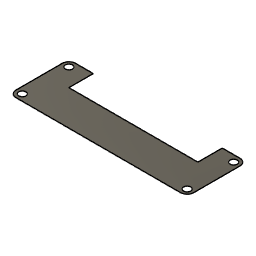
AppleFootToMultiPurposeHolder v1 (Autodesk Fusion 360 design; units mm, degrees)
Autodesk Fusion 360 part; units mm, degrees
sketch "Sketch1" plane through (0, 0, 0) normal (0, 0, 1) x (1, 0, 0)
  line L0 (0, 0) -> (55, 0) construction
  line L1 (0, 0) -> (-55, 0) construction
  circle A0 centre (-57.5, 0) radius 2.5
  circle A1 centre (57.5, 0) radius 2.5
  line L2 (-57.5, -2.5) -> (-57.5, -30) construction
  line L3 (57.5, -2.5) -> (57.5, -30) construction
  circle A2 centre (57.5, -32.5) radius 2.5
  circle A3 centre (-57.5, -32.5) radius 2.5
  circle A4 centre (57.5, 0) radius 4.5
  circle A5 centre (57.5, -32.5) radius 4.5
  circle A6 centre (-57.5, -32.5) radius 4.5
  circle A7 centre (-57.5, 0) radius 4.5
  line L4 (-57.5, 4.5) -> (57.5, 4.5)
  line L5 (62, 0) -> (62, -32.5)
  line L6 (57.5, -37) -> (-57.5, -37)
  line L7 (-62, -32.5) -> (-62, 0)
  line L8 (45, -12.5) -> (-45, -12.5)
  line L9 (-45, -12.5) -> (-45, 12.5)
  line L10 (-45, 12.5) -> (45, 12.5)
  line L11 (45, 12.5) -> (45, -12.5)
  line L12 (45, -12.5) -> (-45, 12.5) construction
  line L13 (-45, -12.5) -> (45, 12.5) construction
  dimension "d1" = 55
  dimension "d2" = 55
  dimension "d4" = 27.5
  dimension "d5" = 27.5
  dimension "d6" = 5
  dimension "d7" = 5
  dimension "d8" = 9
  dimension "d9" = 9
  dimension "d10" = 9
  dimension "d11" = 9
  dimension "d12" = 90
  dimension "d13" = 25
  constraint coincident L0.start L1.start
  constraint horizontal L0
  constraint parallel L0 L1
  constraint coincident L1.end A0
  constraint coincident L0.end A1
  constraint coincident A0 L2.start
  constraint vertical L2
  constraint coincident A1 L3.start
  constraint perpendicular L0 L3
  constraint coincident L3.end A2
  constraint coincident L2.end A3
  constraint concentric A1 A4
  constraint concentric A2 A5
  constraint concentric A3 A6
  constraint concentric A0 A7
  constraint coincident A7 L4.start
  constraint coincident A4 L4.end
  constraint tangent A4 L4
  constraint horizontal L4
  constraint coincident A4 L5.start
  constraint coincident A5 L5.end
  constraint tangent A5 L5
  constraint perpendicular L4 L5
  constraint coincident A5 L6.start
  constraint coincident A6 L6.end
  constraint tangent A6 L6
  constraint perpendicular L5 L6
  constraint coincident A6 L7.start
  constraint coincident A7 L7.end
  constraint tangent A7 L7
  constraint perpendicular L6 L7
  constraint horizontal L8
  constraint perpendicular L8 L9
  constraint parallel L8 L10
  constraint parallel L9 L11
  constraint coincident L12 L0.start
  constraint coincident L13 L0.start
  measures "d1" distance of L0.start L0.end
  measures "d2" distance of L0.start L1.end
  measures "d4" distance of L2.start L2.end
  measures "d5" distance of L3.start L3.end
  measures "d6" diameter of A2
  measures "d7" diameter of A3
  measures "d8" diameter of A4
  measures "d9" diameter of A5
  measures "d10" diameter of A6
  measures "d11" diameter of A7
  measures "d12" distance of L9.end L10.end
  measures "d13" distance of L8.end L9.end
extrude "Extrude1" add sketch "Sketch1" along normal blind 0.2 contours A4 | A4 A5 A6 A7 L4 L5 L6 L7 L8 L9 L11 | A5 | A6 | A7
equation "d1 = ( 110 / 2 ) * 1 mm"
equation "d2 = ( 110 / 2 ) * 1 mm"
